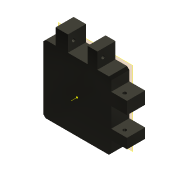
# Autodesk Inventor part: 00_XY_stage-CHUO_SEIKI_LD-647-R1-Middle
Saved by Autodesk Inventor 2019 (Build 230136000, 136)
## iProperties
Created: 2019-05-02
Part Number: 00_XY_stage-CHUO_SEIKI_LD-647-R1-Middle
Material: Generic
Document SubType Name: Modeling
Designer: diederichbenedict
Density: 1 g/cm^3
Appearance: Gunmetal
Author: diederichbenedict
Autodesk Inventor part; units mm, degrees
ref_plane "YZ Plane" through (0, 0, 0) normal (1, 0, 0) x (0, 1, 0)
ref_plane "XZ Plane" through (0, 0, 0) normal (0, 1, 0) x (-1, 0, 0)
ref_plane "XY Plane" through (0, 0, 0) normal (0, 0, 1) x (1, 0, 0)
ref_plane "Work Plane1" through (0, 0, 0) normal (0, 0, 1) x (1, 0, 0)
sketch "Sketch1" plane through (0, 0, 0) normal (0, 0, 1) x (1, 0, 0)
  circle A0 centre (17.5, 17.5) radius 1.95 projected
  circle A1 centre (17.5, -17.5) radius 1.95 projected
  circle A2 centre (-17.5, -17.5) radius 1.95 projected
  circle A3 centre (-17.5, 17.5) radius 1.95 projected
  circle A4 centre (0, 0) radius 7.5 projected
  line L0 (-30, 28) -> (-28, 30) projected
  line L1 (-30, -28) -> (-30, 28) projected
  line L2 (-28, -30) -> (-30, -28) projected
  line L3 (28, -30) -> (-28, -30) projected
  line L4 (30, -28) -> (28, -30) projected
  line L5 (30, 28) -> (30, -28) projected
  line L6 (28, 30) -> (30, 28) projected
  line L7 (-28, 30) -> (28, 30) projected
  circle A5 centre (25, 25) radius 2.325 projected
  circle A6 centre (-25, -25) radius 2.325 projected
  circle A7 centre (25, -25) radius 2.325 projected
  circle A8 centre (-25, 25) radius 2.325 projected
extrude "Extrusion1" add sketch "Sketch1" along normal blind 16 contours A0 | A1 | A2 | A3 | A4 | L0 L7 L6 L5 L4 L3 L2 L1 | A5 | A6 | A7 | A8
sketch "Sketch2" plane through (0, 0, 16) normal (0, 0, 1) x (1, 0, 0)
  point P0 (0, 0)
sketch "Sketch3" plane through (30, -28, 0) normal (1, 0, 0) x (0, 0, -1)
  line L0 (0, 56) -> (0, 0) projected
  line L1 (0, 56) -> (-16, 56) projected
  line L2 (-16, 0) -> (-16, 56) projected
  line L3 (0, 0) -> (-16, 0) projected
  line L4 (-16, 0) -> (-16, 56) projected
  line L5 (0, 47.2331) -> (-16, 47.2331)
  line L6 (-16, 47.2331) -> (-16, 36.3051)
  line L7 (-16, 36.3051) -> (0, 36.3051)
  line L8 (0, 36.3051) -> (0, 47.2331)
  line L9 (0, 56) -> (0, 0) projected
  line L10 (0, 10.2066) -> (-16, 10.2066)
  line L11 (-16, 10.2066) -> (-16, 18.9489)
  line L12 (-16, 18.9489) -> (0, 18.9489)
  line L13 (0, 18.9489) -> (0, 10.2066)
  point P0 (0, 28)
  constraints: 16 end point, 4 parallel, 4 point on line, 2 horizontal, 2 perpendicular
extrude "Extrusion2" add sketch "Sketch3" along normal blind 14 contours L0 L7 L2 L5 | L0 L10 L2 L12
sketch "Sketch4" plane through (30, 19.2331, 16) normal (0, 1, 0) x (1, 0, 0)
  line L0 (0, 0) -> (0, 16) projected
  line L1 (0, 0) -> (14, 0) projected
  line L2 (14, 16) -> (14, 0) projected
  line L3 (0, 16) -> (14, 16) projected
  circle A0 centre (7, 5) radius 1.5
  point P0 (-30, 16)
  dimension "d4" = 3
  constraints: 1 centre point
  measures "d4" diameter of A0
extrude "Extrusion3" cut sketch "Sketch4" against normal through all contours A0
pattern_circular "Circular Pattern1" count 2 over 90 about axis through (0, 0, 0) along (0, 0, 1) of "Extrusion2", "Extrusion3"
body "Solid1"
